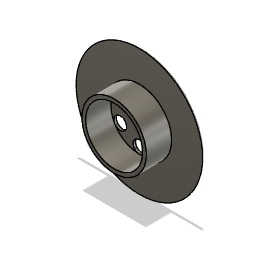
Tapa placard mami (Autodesk Fusion 360 design; units mm, degrees)
Autodesk Fusion 360 part; units mm, degrees
sketch "Sketch1" plane through (0, 0, 0) normal (0, 0, 1) x (1, 0, 0)
  circle A0 centre (0, 0) radius 25
  circle A1 centre (0, 0) radius 12.75
  circle A2 centre (0, 8.75) radius 2.5
  circle A3 centre (-7.5777, 4.375) radius 2.5
  circle A4 centre (-7.5777, -4.375) radius 2.5
  circle A5 centre (0, -8.75) radius 2.5
  circle A6 centre (7.5777, -4.375) radius 2.5
  circle A7 centre (7.5777, 4.375) radius 2.5
  circle A8 centre (0, 0) radius 2.5
  line L0 (0, 0) -> (0, 2.5) construction
  line L1 (0, 2.5) -> (0, 6.25) construction
  line L2 (0, 6.25) -> (0, 11.25) construction
  circle A9 centre (0, 0) radius 11.25
  dimension "d1" = 50
  dimension "d2" = 25.5
  dimension "d3" = 5
  dimension "d5" = 360
  dimension "d7" = 5
  dimension "d11" = 1.5
  constraint coincident A0.centre A1.centre
  constraint concentric A0 A1
  constraint vertical L0
  constraint coincident A2.centre L0
  constraint concentric A1 A8
  constraint coincident A8 L0.end
  constraint coincident A2 L1.end
  constraint coincident A2 L2.end
  constraint vertical L2
  constraint vertical L1
  constraint concentric A1 A9
  constraint tangent A2 A9
  measures "d1" diameter of A0
  measures "d2" diameter of A1
  measures "d3" diameter of A2
  measures "d7" diameter of A8
  measures "d11" distance of A1 A9
extrude "Extrude1" add sketch "Sketch1" against normal blind 1 contours A0 | A1 | A9
extrude "Extrude2" add sketch "Sketch1" along normal blind 10 contours A1
fillet "Fillet1" radius 1 1 edges at (-23.3082, 9.0404, -1)
named bodies: "Coso placard mami"
